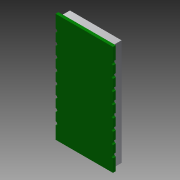
# Autodesk Inventor part: Radio
Saved by Autodesk Inventor 2015 SP1 (Build 190203100, 203)
## iProperties
Created: 2015-10-19
Part Number: Radio
Material: Generic
Document SubType Name: Modeling
Designer: Kartikye
Density: 1 g/cm^3
Appearance: Default
Author: Kartikye
Autodesk Inventor part; units mm, degrees
ref_plane "YZ Plane" through (0, 0, 0) normal (1, 0, 0) x (0, 1, 0)
ref_plane "XZ Plane" through (0, 0, 0) normal (0, 1, 0) x (-1, 0, 0)
ref_plane "XY Plane" through (0, 0, 0) normal (0, 0, 1) x (1, 0, 0)
sketch "Sketch1" plane through (0, 0, 0) normal (0, 1, 0) x (-1, 0, 0)
  line L0 (-10, 19) -> (10, 19)
  line L1 (10, 19) -> (10, -19)
  line L2 (10, -19) -> (-10, -19)
  line L3 (-10, -19) -> (-10, 19)
  line L4 (-10, 19) -> (10, -19) construction
  line L5 (10, 19) -> (-10, -19) construction
  circle A0 centre (10, 14) radius 0.6
  circle A1 centre (10, 10) radius 0.6
  circle A2 centre (10, 6) radius 0.6
  circle A3 centre (10, 2) radius 0.6
  circle A4 centre (10, -2) radius 0.6
  circle A5 centre (10, -6) radius 0.6
  circle A6 centre (10, -10) radius 0.6
  circle A7 centre (10, -14) radius 0.6
  circle A8 centre (-10, 14) radius 0.6
  circle A9 centre (-10, 10) radius 0.6
  circle A10 centre (-10, 6) radius 0.6
  circle A11 centre (-10, 2) radius 0.6
  circle A12 centre (-10, -2) radius 0.6
  circle A13 centre (-10, -6) radius 0.6
  circle A14 centre (-9.9999, -10) radius 0.6
  circle A15 centre (-9.9999, -14) radius 0.6
  point P0 (0, 0)
  dimension "d0" = 20
  dimension "d1" = 38
  dimension "d2" = 1.2
  dimension "d3" = 0
  dimension "d4" = 5
  dimension "d5" = 1.2
  dimension "d6" = 1.2
  dimension "d7" = 0
  dimension "d8" = 0
  dimension "d9" = 4
  dimension "d10" = 4
  dimension "d11" = 1.2
  dimension "d13" = 1.2
  dimension "d14" = 1.2
  dimension "d15" = 0
  dimension "d16" = 0
  dimension "d17" = 0
  dimension "d18" = 4
  dimension "d19" = 4
  dimension "d20" = 4
  dimension "d22" = 1.2
  dimension "d23" = 0
  dimension "d24" = 4
  dimension "d25" = 1.2
  dimension "d26" = 0
  dimension "d27" = 4
  dimension "d28" = 1.2
  dimension "d29" = 1.2
  dimension "d30" = 1.2
  dimension "d31" = 4
  dimension "d32" = 4
  dimension "d33" = 1.2
  dimension "d34" = 4
  dimension "d35" = 5
  dimension "d36" = 0
  dimension "d37" = 1.2
  dimension "d38" = 1.2
  dimension "d39" = 1.2
  dimension "d40" = 4
  dimension "d41" = 4
  dimension "d42" = 1.2
  dimension "d43" = 4
  dimension "d44" = 5
  dimension "d45" = 0
  dimension "d46" = 4
  constraints: 16 centre point, 12 end point, 2 midpoint, 2 parallel, 1 horizontal, 1 perpendicular
  measures "d0" distance of L1.end L2.end
  measures "d1" distance of L0.end L1.end
  measures "d2" diameter of A0
  measures "d3" distance from line of L1 A0.centre
  measures "d4" distance from line of L0 A0.centre
  measures "d5" diameter of A1
  measures "d6" diameter of A2
  measures "d7" distance from line of A1.centre L1
  measures "d8" distance from line of A2.centre L1
  measures "d9" distance of A1.centre A0.centre
  measures "d10" distance of A2.centre A1.centre
  measures "d11" diameter of A3
  measures "d13" diameter of A4
  measures "d14" diameter of A5
  measures "d15" distance from line of A3.centre L1
  measures "d16" distance from line of A4.centre L1
  measures "d17" distance from line of A5.centre L1
  measures "d18" distance of A3.centre A2.centre
  measures "d19" distance of A4.centre A3.centre
  measures "d20" distance of A5.centre A4.centre
  measures "d22" diameter of A6
  measures "d23" distance from line of A6.centre L1
  measures "d24" distance of A6.centre A5.centre
  measures "d25" diameter of A7
  measures "d26" distance from line of A7.centre L1
  measures "d27" distance of A7.centre A6.centre
  measures "d28" diameter of A8
  measures "d29" diameter of A9
  measures "d30" diameter of A10
  measures "d31" distance of A9.centre A8.centre
  measures "d32" distance of A10.centre A9.centre
  measures "d33" diameter of A11
  measures "d34" distance of A11.centre A10.centre
  measures "d35" distance from line of L0 A8.centre
  measures "d36" distance from line of L3 A8.centre
  measures "d37" diameter of A12
  measures "d38" diameter of A13
  measures "d39" diameter of A14
  measures "d40" distance of A13.centre A12.centre
  measures "d41" distance of A14.centre A13.centre
  measures "d42" diameter of A15
  measures "d43" distance of A15.centre A14.centre
  measures "d44" distance from line of L2 A15.centre
  measures "d45" distance from line of A12.centre L3
  measures "d46" distance of A12.centre A11.centre
extrude "Extrusion1" add sketch "Sketch1" along normal blind 1 contours L0 L1 A0 A1 A2 A3 A4 A5 A6 A7 L2 L3 A15 A14 A13 A12 A11 A10 A9 A8 | A8 L3 | L1 A0 | A9 L3 | L1 A1 | A10 L3 | L1 A2 | A11 L3 | L1 A3 | A12 L3 | L1 A4 | A13 L3 | L1 A5 | A14 L3 | L1 A6 | A15 L3 | L1 A7 picked at (-9.7546, 14.1247) picked at (9.9071, 13.8229) picked at (-9.7546, 10.1247) picked at (9.9071, 9.8229) picked at (-9.7991, 6.1197) picked at (9.6869, 6.1942) picked at (-9.7124, 2.1099) picked at (9.9521, 1.8058) picked at (-9.8308, -1.8486) picked at (9.9521, -2.1942) picked at (-9.7863, -5.8436) picked at (9.6325, -6.0264) picked at (-9.8, -10) picked at (9.7266, -9.8332) picked at (-9.8, -14) picked at (9.7266, -13.8332)
sketch "Sketch2" plane through (0, 1, 0) normal (0, 1, 0) x (1, 0, 0)
  line L0 (-10, 19) -> (10, 19)
  line L1 (10, 19) -> (10, -19)
  line L2 (10, -19) -> (-10, -19)
  line L3 (-10, -19) -> (-10, 19)
  line L4 (-10, 19) -> (10, -19) construction
  line L5 (10, 19) -> (-10, -19) construction
  circle A0 centre (10, 14) radius 0.6
  circle A1 centre (10, 10) radius 0.6
  circle A2 centre (10, 6) radius 0.6
  circle A3 centre (10, 2) radius 0.6
  circle A4 centre (10, -2) radius 0.6
  circle A5 centre (10, -6) radius 0.6
  circle A6 centre (10, -10) radius 0.6
  circle A7 centre (10, -14) radius 0.6
  circle A8 centre (-10, 14) radius 0.6
  circle A9 centre (-10, 10) radius 0.6
  circle A10 centre (-10, 6) radius 0.6
  circle A11 centre (-10, 2) radius 0.6
  circle A12 centre (-10, -2) radius 0.6
  circle A13 centre (-10, -6) radius 0.6
  circle A14 centre (-9.9999, -10) radius 0.6
  circle A15 centre (-9.9999, -14) radius 0.6
  point P0 (0, 0)
  point P1 (0, 0)
  dimension "d49" = 20
  dimension "d50" = 38
  dimension "d51" = 1.2
  dimension "d52" = 0
  dimension "d53" = 5
  dimension "d54" = 1.2
  dimension "d55" = 1.2
  dimension "d56" = 0
  dimension "d57" = 0
  dimension "d58" = 4
  dimension "d59" = 4
  dimension "d60" = 1.2
  dimension "d61" = 1.2
  dimension "d62" = 1.2
  dimension "d63" = 0
  dimension "d64" = 0
  dimension "d65" = 0
  dimension "d66" = 4
  dimension "d67" = 4
  dimension "d68" = 4
  dimension "d69" = 1.2
  dimension "d70" = 0
  dimension "d71" = 4
  dimension "d72" = 1.2
  dimension "d73" = 0
  dimension "d74" = 4
  dimension "d75" = 1.2
  dimension "d76" = 1.2
  dimension "d77" = 1.2
  dimension "d78" = 4
  dimension "d79" = 4
  dimension "d80" = 1.2
  dimension "d81" = 4
  dimension "d82" = 5
  dimension "d83" = 0
  dimension "d84" = 1.2
  dimension "d85" = 1.2
  dimension "d86" = 1.2
  dimension "d87" = 4
  dimension "d88" = 4
  dimension "d89" = 1.2
  dimension "d90" = 4
  dimension "d91" = 5
  dimension "d92" = 0
  dimension "d93" = 4
  constraints: 16 centre point, 12 end point, 2 midpoint, 2 parallel, 1 horizontal, 1 perpendicular
  measures "d49" distance of L1.end L2.end
  measures "d50" distance of L0.end L1.end
  measures "d51" diameter of A0
  measures "d52" distance from line of L1 A0.centre
  measures "d53" distance from line of L0 A0.centre
  measures "d54" diameter of A1
  measures "d55" diameter of A2
  measures "d56" distance from line of A1.centre L1
  measures "d57" distance from line of A2.centre L1
  measures "d58" distance of A1.centre A0.centre
  measures "d59" distance of A2.centre A1.centre
  measures "d60" diameter of A3
  measures "d61" diameter of A4
  measures "d62" diameter of A5
  measures "d63" distance from line of A3.centre L1
  measures "d64" distance from line of A4.centre L1
  measures "d65" distance from line of A5.centre L1
  measures "d66" distance of A3.centre A2.centre
  measures "d67" distance of A4.centre A3.centre
  measures "d68" distance of A5.centre A4.centre
  measures "d69" diameter of A6
  measures "d70" distance from line of A6.centre L1
  measures "d71" distance of A6.centre A5.centre
  measures "d72" diameter of A7
  measures "d73" distance from line of A7.centre L1
  measures "d74" distance of A7.centre A6.centre
  measures "d75" diameter of A8
  measures "d76" diameter of A9
  measures "d77" diameter of A10
  measures "d78" distance of A9.centre A8.centre
  measures "d79" distance of A10.centre A9.centre
  measures "d80" diameter of A11
  measures "d81" distance of A11.centre A10.centre
  measures "d82" distance from line of L0 A8.centre
  measures "d83" distance from line of L3 A8.centre
  measures "d84" diameter of A12
  measures "d85" diameter of A13
  measures "d86" diameter of A14
  measures "d87" distance of A13.centre A12.centre
  measures "d88" distance of A14.centre A13.centre
  measures "d89" diameter of A15
  measures "d90" distance of A15.centre A14.centre
  measures "d91" distance from line of L2 A15.centre
  measures "d92" distance from line of A12.centre L3
  measures "d93" distance of A12.centre A11.centre
extrude "Extrusion2" cut sketch "Sketch2" against normal blind 1 contours A8 L3 | L3 A8 | A0 L1 | L1 A0 | A9 L3 | L3 A9 | A1 L1 | L1 A1 | A10 L3 | L3 A10 | A2 L1 | L1 A2 | A11 L3 | L3 A11 | A3 L1 | L1 A3 | A12 L3 | L3 A12 | A4 L1 | L1 A4 | A13 L3 | L3 A13 | A5 L1 | L1 A5 | A14 L3 | L3 A14 | A6 L1 | L1 A6 | A15 L3 | L3 A15 | A7 L1 | L1 A7
sketch "Sketch3" plane through (0, 1, 0) normal (0, 1, 0) x (1, 0, 0)
  line L0 (-9, -18.5) -> (9, -18.5)
  line L1 (9, -18.5) -> (9, 18.5)
  line L2 (9, 18.5) -> (-9, 18.5)
  line L3 (-9, 18.5) -> (-9, -18.5)
  line L4 (-9, -18.5) -> (9, 18.5) construction
  line L5 (9, -18.5) -> (-9, 18.5) construction
  point P0 (0, 0)
  dimension "d96" = 37
  constraints: 12 end point, 2 midpoint, 2 parallel, 1 horizontal, 1 perpendicular
  measures "d96" distance of L1.end L0.end
extrude "Extrusion3" add sketch "Sketch3" along normal blind 3
body "Solid1"
